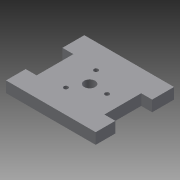
# Autodesk Inventor part: motor holder
Saved by Autodesk Inventor 2015 (Build 190159000, 159)
## iProperties
Created: 2015-03-03
Part Number: motor holder
Material: Generic
Document SubType Name: Modeling
Designer: Qiuyang
Density: 1 g/cm^3
Appearance: Default
Author: Qiuyang
Autodesk Inventor part; units mm, degrees
ref_plane "YZ Plane" through (0, 0, 0) normal (1, 0, 0) x (0, 1, 0)
ref_plane "XZ Plane" through (0, 0, 0) normal (0, 1, 0) x (-1, 0, 0)
ref_plane "XY Plane" through (0, 0, 0) normal (0, 0, 1) x (1, 0, 0)
sketch "Sketch1" plane through (0, 0, 0) normal (0, 1, 0) x (-1, 0, 0)
  line L0 (0, 0) -> (-44.45, 0)
  line L1 (-44.45, 0) -> (-44.45, -47.5996)
  line L2 (-44.45, -47.5996) -> (0, -47.5996)
  line L3 (0, -47.5996) -> (0, 0)
  dimension "d0" = 44.45
  dimension "d1" = 47.5996
  constraints: 8 end point, 2 parallel, 1 horizontal, 1 perpendicular
  measures "d0" distance of L2.end L1.end
  measures "d1" distance of L1.end L0.end
extrude "Extrusion1" add sketch "Sketch1" along normal blind 6.35
sketch "Sketch2" plane through (0, 6.35, 0) normal (0, 1, 0) x (1, 0, 0)
  line L0 (0, 47.5996) -> (0, 0) projected
  line L1 (0, 12.7) -> (6.35, 12.7)
  line L2 (6.35, 12.7) -> (6.35, 34.036)
  line L3 (6.35, 34.036) -> (0, 34.036)
  line L4 (0, 34.036) -> (0, 12.7)
  line L5 (44.45, 0) -> (44.45, 47.5996) projected
  line L6 (44.45, 12.7) -> (38.1, 12.7)
  line L7 (38.1, 12.7) -> (38.1, 34.036)
  line L8 (38.1, 34.036) -> (44.45, 34.036)
  line L9 (44.45, 34.036) -> (44.45, 12.7)
  dimension "d4" = 6.35
  dimension "d5" = 21.336
  dimension "d6" = 6.35
  constraints: 16 end point, 4 parallel, 3 point on line, 2 horizontal, 2 perpendicular
  measures "d4" distance of L3.end L2.end
  measures "d5" distance of L2.end L1.end
  measures "d6" distance of L7.end L8.end
extrude "Extrusion2" cut sketch "Sketch2" against normal blind 6.35
sketch "Sketch3" plane through (0, 6.35, 0) normal (0, 1, 0) x (1, 0, 0)
  circle A0 centre (22.225, 23.7998) radius 3.175
  circle A1 centre (32.3088, 23.7998) radius 1.27
  circle A2 centre (17.1831, 32.5326) radius 1.27
  circle A3 centre (17.1831, 15.067) radius 1.27
  point P0 (0, 0)
  dimension "d9" = 6.35
  dimension "d10" = 2.54
  dimension "d13" = 360
  constraints: 4 centre point, 7 other
  measures "d9" diameter of A0
  measures "d10" diameter of A1
extrude "Extrusion3" cut sketch "Sketch3" against normal blind 6.35
sketch "Sketch4" plane through (0, 6.35, 0) normal (0, 1, 0) x (1, 0, 0)
  line L0 (44.45, 47.5996) -> (48.26, 47.5996)
  line L1 (48.26, 47.5996) -> (48.26, 0)
  line L2 (48.26, 0) -> (44.45, 0)
  line L3 (44.45, 0) -> (44.45, 47.5996)
  line L4 (0, 47.5996) -> (-3.81, 47.5996)
  line L5 (-3.81, 47.5996) -> (-3.81, 0)
  line L6 (-3.81, 0) -> (0, 0)
  line L7 (0, 0) -> (0, 47.5996)
  line L8 (0, 12.7) -> (6.35, 12.7) projected
  line L9 (6.35, 34.036) -> (2.54, 34.036)
  line L10 (2.54, 34.036) -> (2.54, 12.7)
  line L11 (2.54, 12.7) -> (6.35, 12.7)
  line L12 (6.35, 12.7) -> (6.35, 34.036)
  line L13 (44.45, 12.7) -> (38.1, 12.7) projected
  line L14 (38.1, 34.036) -> (41.91, 34.036)
  line L15 (41.91, 34.036) -> (41.91, 12.7)
  line L16 (41.91, 12.7) -> (38.1, 12.7)
  line L17 (38.1, 12.7) -> (38.1, 34.036)
  point P0 (0, 0)
  dimension "d17" = 3.81
  dimension "d18" = 3.81
  dimension "d19" = 3.81
  dimension "d20" = 3.81
  constraints: 32 end point, 8 parallel, 4 horizontal, 4 perpendicular, 3 point on line
  measures "d17" distance of L1.end L2.end
  measures "d18" distance of L6.end L5.end
  measures "d19" distance of L11.end L10.end
  measures "d20" distance of L15.end L16.end
extrude "Extrusion4" add sketch "Sketch4" against normal blind 6.35
sketch "Sketch5" plane through (0, 6.35, 0) normal (0, 1, 0) x (1, 0, 0)
  line L0 (-3.81, 0) -> (-3.81, 47.5996) projected
  line L1 (0, 34.036) -> (-3.81, 34.036)
  line L2 (-3.81, 34.036) -> (-3.81, 12.7)
  line L3 (-3.81, 12.7) -> (0, 12.7)
  line L4 (0, 12.7) -> (0, 34.036)
  line L5 (48.26, 47.5996) -> (48.26, 0) projected
  line L6 (44.45, 34.036) -> (48.26, 34.036)
  line L7 (48.26, 34.036) -> (48.26, 12.7)
  line L8 (48.26, 12.7) -> (44.45, 12.7)
  line L9 (44.45, 12.7) -> (44.45, 34.036)
  point P0 (0, 0)
  constraints: 16 end point, 4 parallel, 3 point on line, 2 horizontal, 2 perpendicular
extrude "Extrusion5" cut sketch "Sketch5" against normal blind 6.35
sketch "Sketch6" plane through (0, 6.35, 0) normal (0, 1, 0) x (1, 0, 0)
  line L0 (48.26, 12.7) -> (48.26, 0) projected
  line L1 (-3.81, 0) -> (48.26, 0)
  line L2 (48.26, 0) -> (48.26, 1.27)
  line L3 (48.26, 1.27) -> (-3.81, 1.27)
  line L4 (-3.81, 1.27) -> (-3.81, 0)
  line L5 (48.26, 47.5996) -> (48.26, 34.036) projected
  line L6 (-3.81, 47.5996) -> (48.26, 47.5996)
  line L7 (48.26, 47.5996) -> (48.26, 46.736)
  line L8 (48.26, 46.736) -> (-3.81, 46.736)
  line L9 (-3.81, 46.736) -> (-3.81, 47.5996)
  point P0 (0, 0)
  dimension "d25" = 1.27
  dimension "d26" = 0.8636
  constraints: 16 end point, 4 parallel, 2 horizontal, 2 perpendicular, 2 point on line
  measures "d25" distance of L2.end L1.end
  measures "d26" distance of L6.end L7.end
extrude "Extrusion6" cut sketch "Sketch6" against normal blind 25.4
body "Solid1"
